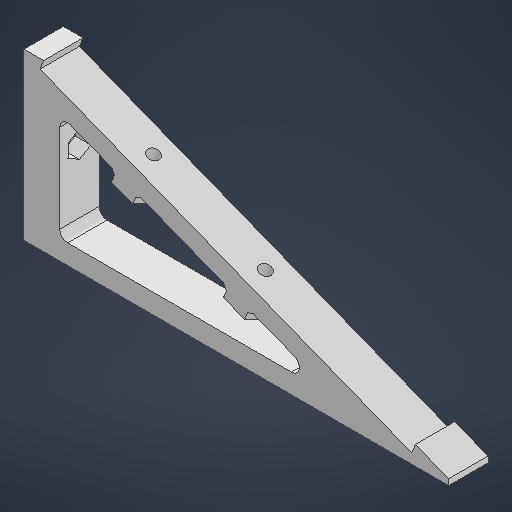
# Autodesk Inventor part: Wall_Stand
Saved by Autodesk Inventor 2026.3 (Build 303398000, 398)
## iProperties
Created: 2026-09-07
Part Number: Wall_Stand
Material: 一般
Document SubType Name: Modeling
Designer: takuya
Density: 1 g/cm^3
Appearance: 既定
Author: takuya
Autodesk Inventor part; units mm, degrees
ref_plane "YZ Plane" through (0, 0, 0) normal (1, 0, 0) x (0, 1, 0)
ref_plane "XZ Plane" through (0, 0, 0) normal (0, 1, 0) x (-1, 0, 0)
ref_plane "XY Plane" through (0, 0, 0) normal (0, 0, 1) x (1, 0, 0)
sketch "スケッチ1" plane through (0, 0, 0) normal (0, 0, 1) x (1, 0, 0)
  line L0 (33, 9) -> (33, -8) projected
  line L1 (33, -8) -> (20, -8) projected
  line L2 (33, 9) -> (33, 34)
  line L3 (33, -8) -> (43, -8)
  line L4 (43, -8) -> (144.5196, -8)
  line L5 (33, 34) -> (38, 34)
  line L6 (38, 34) -> (37.083, 31.6743)
  line L7 (38, 34) -> (37.083, 31.6743)
  line L8 (37.083, 31.6743) -> (131.3636, -5.5)
  line L9 (131.3636, -5.5) -> (132.2807, -3.1743)
  line L10 (132.2807, -3.1743) -> (38, 34)
  line L11 (131.3636, -5.5) -> (131.3636, -8)
  line L12 (132.2807, -3.1743) -> (144.5196, -8)
  line L13 (140.7153, -6.5) -> (140.7153, -8)
  line L14 (37.083, 31.6743) -> (37.083, -8)
  line L15 (42.083, 24.3282) -> (42.083, -3)
  line L16 (42.083, -3) -> (111.3921, -3)
  line L17 (111.3921, -3) -> (42.083, 24.3282)
  point P0 (0, 0)
  point P1 (30, 9)
  dimension "d0" = 25
  dimension "d1" = 10
  dimension "d2" = 5
  dimension "d4" = 2.5
  dimension "d8" = 2.5
  dimension "d9" = 1.5
  dimension "d10" = 5
  dimension "d11" = 5
  dimension "d12" = 5
  constraints: 32 end point, 5 point on line, 4 parallel, 4 perpendicular, 2 horizontal, 2 vertical, 1 collinear, 2 other
  measures "d0" distance of L0.start L2.end
  measures "d1" distance of L0.end L3.end
  measures "d2" distance of L2.end L5.end
  measures "d4" distance of L5.end L6.end
  measures "d8" distance of L8.end L11.end
  measures "d9" distance of L13.start L13.end
  measures "d10" distance between parallel lines of L8 L17
  measures "d11" distance between parallel lines of L4 L16
  measures "d12" distance between parallel lines of L14 L15
extrude "押し出し1" add sketch "スケッチ1" against normal blind 10 contours L2 L5 L6 L14 L3 L0 | L14 L8 L11 L4 L3 | L12 L13 L4 L11 L9
fillet "フィレット1" radius 2 3 edges at (42.083, 24.3282, -5) (42.083, -3, -5) (111.3921, -3, -5)
sketch "スケッチ2" plane through (33, -8, 0) normal (-1, 0, 0) x (0, 0, 1)
  line L0 (0, 42) -> (0, 0) projected
  line L1 (0, 42) -> (-10, 42) projected
  line L2 (-10, 0) -> (-10, 42) projected
  line L3 (0, 0) -> (-10, 0) projected
  line L4 (0, 17) -> (0, 0) projected
  line L5 (-198, 0) -> (0, 0) projected
  line L6 (-198, 17) -> (-198, 0) projected
  line L7 (-198, 17) -> (0, 17) projected
  line L8 (-8.85, 9) -> (-1.15, 9)
  line L9 (-1.15, 9) -> (-1.15, 5)
  line L10 (-1.15, 5) -> (-8.85, 5)
  line L11 (-8.85, 5) -> (-8.85, 9)
  line L12 (-10, 5) -> (0, 5) projected
  line L13 (0, 5) -> (-10, 5) projected
  line L14 (-8.75, 5) -> (-1.25, 5) projected
  line L15 (-8.75, 9) -> (-8.75, 5) projected
  line L16 (-1.25, 5) -> (-1.25, 9) projected
  line L17 (-8.75, 9) -> (-1.25, 9) projected
  line L18 (-189.25, 9) -> (-196.75, 9) projected
  line L19 (-196.75, 9) -> (-196.75, 5) projected
  line L20 (-196.75, 5) -> (-189.25, 5) projected
  line L21 (-189.25, 5) -> (-189.25, 9) projected
  point P0 (0, 8)
  point P1 (-5, 9)
  point P2 (-5, 42)
  point P3 (-5, 5)
  point P4 (-8.65, 5)
  point P5 (-1.35, 5)
  dimension "d16" = 7.7
  dimension "d17" = 4
  constraints: 8 end point, 4 midpoint, 2 parallel, 1 horizontal, 1 perpendicular, 1 vertical alignment
  measures "d16" distance of L8.start L8.end
  measures "d17" distance of L10.end L8.start
extrude "押し出し2" cut sketch "スケッチ2" against normal blind 7.7 contours L10 L16 L8 L9 | L10 L15 L8 L16 | L11 L8 L15 L10
sketch "スケッチ3" plane through (33, -8, 0) normal (-1, 0, 0) x (0, 0, 1)
  line L0 (-1.15, 5) -> (-8.85, 5) projected
  line L1 (-8.85, 5) -> (-8.85, 9) projected
  line L2 (-8.85, 9) -> (-1.15, 9) projected
  line L3 (-1.15, 9) -> (-1.15, 5) projected
  line L4 (0, 42) -> (0, 0) projected
  line L5 (0, 42) -> (-10, 42) projected
  line L6 (-10, 0) -> (-10, 42) projected
  line L7 (0, 0) -> (-10, 0) projected
  circle A0 centre (-15, 23.1949) radius 1.5
  line L8 (-15, 23.1949) -> (0, 23.1949)
  line L9 (0, 42) -> (0, 0) projected
  circle A1 centre (-5, 23.1949) radius 1.5
  point P0 (0, 8)
  dimension "d20" = 3
  constraints: 2 centre point, 2 end point, 2 point on line, 1 perpendicular, 2 other
  measures "d20" diameter of A1
extrude "押し出し3" cut sketch "スケッチ3" against normal blind 10 contours A1 L8 | L8 A1
sketch "スケッチ4" plane through (101.601, 0.8606, -10) normal (-0.3668097, -0.930296, 0) x (0.930296, -0.3668097, 0)
  circle A0 centre (-45.7793, 5) radius 1.5
  circle A1 centre (-15.2598, 5) radius 1.5
  point P0 (-94.2033, 10)
  constraints: 2 centre point, 4 other
extrude "押し出し4" cut sketch "スケッチ4" against normal blind 10
sketch "スケッチ5" plane through (33, -8, 0) normal (0, -1, 0) x (1, 0, 0)
  circle A0 centre (3.9, -5) radius 1.5
  point P0 (-33, 0)
  constraints: 1 centre point, 2 other
extrude "押し出し5" cut sketch "スケッチ5" against normal up to surface (9 mm away)
sketch "スケッチ6" plane through (33, -8, 0) normal (0, -1, 0) x (1, 0, 0)
  circle A0 centre (3.9, -5) radius 1.5 projected
  line L0 (0, 0) -> (107.7153, 0) projected
  line L1 (0, 0) -> (0, -10) projected
  line L2 (107.7153, -10) -> (0, -10) projected
  line L3 (107.7153, 0) -> (107.7153, -10) projected
  circle A1 centre (3.9, -5) radius 3
  point P0 (-33, 0)
  dimension "d27" = 6
  constraints: 1 centre point, 1 coincident
  measures "d27" diameter of A1
extrude "押し出し6" cut sketch "スケッチ6" against normal blind 3 contours A0 | A1
sketch "スケッチ7" plane through (101.601, 0.8606, -10) normal (-0.3668097, -0.930296, 0) x (0.930296, -0.3668097, 0)
  circle A0 centre (-45.7793, 5) radius 1.5 projected
  circle A1 centre (-15.2598, 5) radius 1.5 projected
  line L0 (30.0212, 10) -> (-71.3236, 10) projected
  line L1 (30.0212, 10) -> (30.0212, 0) projected
  line L2 (-71.3236, 0) -> (30.0212, 0) projected
  line L3 (-71.3236, 10) -> (-71.3236, 0) projected
  line L4 (-44.1002, 7.8973) -> (-42.4307, 4.9945)
  line L5 (-42.4307, 4.9945) -> (-44.1097, 2.0973)
  line L6 (-44.1097, 2.0973) -> (-47.4584, 2.1027)
  line L7 (-47.4584, 2.1027) -> (-49.1279, 5.0055)
  line L8 (-49.1279, 5.0055) -> (-47.4489, 7.9027)
  line L9 (-47.4489, 7.9027) -> (-44.1002, 7.8973)
  line L10 (-13.6143, 7.85) -> (-11.9689, 5)
  line L11 (-11.9689, 5) -> (-13.6143, 2.15)
  line L12 (-13.6143, 2.15) -> (-16.9052, 2.15)
  line L13 (-16.9052, 2.15) -> (-18.5507, 5)
  line L14 (-18.5507, 5) -> (-16.9052, 7.85)
  line L15 (-16.9052, 7.85) -> (-13.6143, 7.85)
  line L16 (-42.8925, 10) -> (-40.0058, 5)
  line L17 (-40.0058, 5) -> (-42.8925, 0)
  line L18 (-42.8925, 0) -> (-48.666, 0)
  line L19 (-48.666, 0) -> (-51.5528, 5)
  line L20 (-51.5528, 5) -> (-48.666, 10)
  line L21 (-48.666, 10) -> (-42.8925, 10)
  line L22 (-12.373, 10) -> (-9.4863, 5)
  line L23 (-9.4863, 5) -> (-12.373, 0)
  line L24 (-12.373, 0) -> (-18.1465, 0)
  line L25 (-18.1465, 0) -> (-21.0333, 5)
  line L26 (-21.0333, 5) -> (-18.1465, 10)
  line L27 (-18.1465, 10) -> (-12.373, 10)
  point P0 (-94.2033, 10)
  point P1 (-15.2598, 7.85)
  point P2 (-45.7745, 7.9)
  point P3 (-45.784, 2.1)
  point P4 (-45.7793, 10)
  point P5 (-15.2598, 10)
  point P6 (-18.1465, 10)
  point P7 (-18.1465, 0)
  point P8 (-12.373, 0)
  point P9 (-12.373, 10)
  point P10 (-48.666, 0)
  point P11 (-42.8925, 0)
  dimension "d30" = 5.7
  dimension "d31" = 5.8
  constraints: 48 end point, 5 midpoint, 4 coincident, 3 point on line, 1 parallel, 52 other
  measures "d30" distance from line of point (-15.26, 7.85) L12
  measures "d31" distance of point (-45.775, 7.9) point (-45.784, 2.1)
extrude "押し出し7" add sketch "スケッチ7" along normal blind 3 contours L22 L23 L2 L25 L26 L0 | L16 L17 L2 L19 L20 L0
chamfer "面取り1" distance 1 angle 45 8 edges at (83.3766, 8.0464, -7.5) (83.3766, 8.0464, -2.5) (91.4332, 4.8697, -7.5) (91.4332, 4.8697, -2.5) (63.041, 16.0645, -2.5) (54.9844, 19.2412, -2.5) (63.041, 16.0645, -7.5) (54.9844, 19.2412, -7.5)
sketch "スケッチ8" plane through (42.083, -1, 0) normal (1, 0, 0) x (0, 0, -1)
  circle A0 centre (5, 16.1949) radius 1.5 construction
  line L0 (5, 19.5435) -> (7.9, 17.8692)
  line L1 (7.9, 17.8692) -> (7.9, 14.5205)
  line L2 (7.9, 14.5205) -> (5, 12.8462)
  line L3 (5, 12.8462) -> (2.1, 14.5205)
  line L4 (2.1, 14.5205) -> (2.1, 17.8692)
  line L5 (2.1, 17.8692) -> (5, 19.5435)
  circle A1 centre (5, 16.1949) radius 1.5 projected
  line L6 (10, 0) -> (0, 0) projected
  line L7 (10, 22.3897) -> (10, 0) projected
  line L8 (0, 22.3897) -> (10, 22.3897) projected
  line L9 (0, 0) -> (0, 22.3897) projected
  point P0 (0, 1)
  dimension "d37" = 5.8
  constraints: 12 end point, 1 coincident, 13 other
  measures "d37" distance between parallel lines of L1 L4
extrude "押し出し8" cut sketch "スケッチ8" against normal blind 4 contours L0 L1 L2 L3 L4 L5
